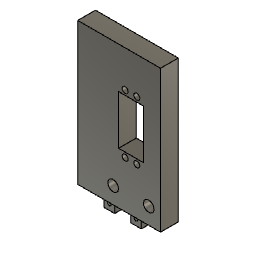
servo_side_stand_2 v20 (Autodesk Fusion 360 design; units mm, degrees)
Autodesk Fusion 360 part; units mm, degrees
note: some values were not read from the file. Set by a fixed rule: which sketch regions a step uses.
sketch "Sketch1" plane through (0, 0, 0) normal (0, 0, 1) x (1, 0, 0)
  line L0 (45, -7.5) -> (-45, -7.5) construction
  line L1 (-45, -7.5) -> (-45, 7.5) construction
  line L2 (-45, 7.5) -> (45, 7.5) construction
  line L3 (45, 7.5) -> (45, -7.5) construction
  line L4 (45, -7.5) -> (-45, 7.5) construction
  line L5 (-45, -7.5) -> (45, 7.5) construction
  line L6 (0, -7.5) -> (45, 7.5) construction
  line L7 (-45, 7.5) -> (0, -7.5) construction
  line L8 (4.5, -3.25) -> (-4.5, -3.25)
  line L9 (-4.5, -3.25) -> (-4.5, 3.25)
  line L10 (-4.5, 3.25) -> (4.5, 3.25)
  line L11 (4.5, 3.25) -> (4.5, -3.25)
  line L12 (4.5, -3.25) -> (-4.5, 3.25) construction
  line L13 (-4.5, -3.25) -> (4.5, 3.25) construction
  line L14 (-27, -3.25) -> (-18, -3.25)
  line L15 (-18, -3.25) -> (-18, 3.25)
  line L16 (-18, 3.25) -> (-27, 3.25)
  line L17 (-27, 3.25) -> (-27, -3.25)
  line L18 (-27, -3.25) -> (-18, 3.25) construction
  line L19 (-18, -3.25) -> (-27, 3.25) construction
  point P0 (22.5, 0)
  point P1 (-22.5, 0)
  dimension "d1" = 90
  dimension "d2" = 15
  dimension "d3" = 9
  dimension "d4" = 9
  dimension "d7" = 6.5
  dimension "d8" = 6.5
  constraint horizontal L0
  constraint perpendicular L0 L1
  constraint parallel L0 L2
  constraint parallel L1 L3
  constraint coincident L4 origin
  constraint coincident L5 origin
  constraint midpoint L0 L6.start
  constraint horizontal L8
  constraint perpendicular L8 L9
  constraint parallel L8 L10
  constraint parallel L9 L11
  constraint coincident L12 origin
  constraint coincident L13 origin
  constraint midpoint L6 P0
  constraint horizontal L14
  constraint perpendicular L14 L15
  constraint parallel L14 L16
  constraint parallel L15 L17
  constraint coincident L18 P1
  constraint coincident L19 P1
  constraint midpoint L7 P1
  measures "d1" distance of L0.start L0.end
  measures "d2" distance of L0.end L1.end
  measures "d3" distance of L14.start L14.end
  measures "d4" distance of L8.start L8.end
  measures "d7" distance of L8.start L10.end
  measures "d8" distance of L14.end L15.end
extrude "Extrude1" add sketch "Sketch1" along normal blind 10 makes body 1 at (-21, 3.25, 3.3333) makes body 2 at (-1.5, 3.25, 3.3333)
sketch "Sketch2" plane through (0, 0, 10) normal (0, 0, 1) x (-1, 0, 0)
  line L0 (45, 7.5) -> (-45, 7.5)
  line L1 (-45, 7.5) -> (-45, -7.5)
  line L2 (-45, -7.5) -> (45, -7.5)
  line L3 (45, -7.5) -> (45, 7.5)
  line L4 (45, 7.5) -> (-45, -7.5) construction
  line L5 (-45, 7.5) -> (45, -7.5) construction
  line L6 (27, -3.25) -> (27, 3.25)
  line L7 (27, 3.25) -> (18, 3.25)
  line L8 (18, 3.25) -> (18, -3.25)
  line L9 (18, -3.25) -> (27, -3.25)
  line L10 (-4.5, -3.25) -> (4.5, -3.25)
  line L11 (4.5, -3.25) -> (4.5, 3.25)
  line L12 (4.5, 3.25) -> (-4.5, 3.25)
  line L13 (-4.5, 3.25) -> (-4.5, -3.25)
  dimension "d11" = 90
  dimension "d12" = 15
  constraint horizontal L0
  constraint perpendicular L0 L1
  constraint parallel L0 L2
  constraint parallel L1 L3
  constraint coincident L4 origin
  constraint coincident L5 origin
  measures "d11" distance of L0.start L0.end
  measures "d12" distance of L0.start L2.end
extrude "Extrude2" add sketch "Sketch2" along normal blind 120 contours L0 L1 L2 L3 | L6 L7 L8 L9 | L10 L11 L12 L13 bodies 1 2
sketch "Sketch3" plane through (0, -7.5, 0) normal (0, -1, 0) x (1, 0, 0)
  line L0 (-45, 10) -> (45, 10)
  line L1 (45, 10) -> (45, 130)
  line L2 (45, 130) -> (-45, 130)
  line L3 (-45, 130) -> (-45, 10)
  line L4 (0, 10) -> (0, 74.4) construction
  line L5 (10.5, 53.65) -> (-10.5, 53.65)
  line L6 (-10.5, 53.65) -> (-10.5, 95.15)
  line L7 (-10.5, 95.15) -> (10.5, 95.15)
  line L8 (10.5, 95.15) -> (10.5, 53.65)
  line L9 (10.5, 53.65) -> (-10.5, 95.15) construction
  line L10 (-10.5, 53.65) -> (10.5, 95.15) construction
  line L11 (10, 49.65) -> (-10, 49.65) construction
  line L12 (-10, 49.65) -> (-10, 99.15) construction
  line L13 (-10, 99.15) -> (10, 99.15) construction
  line L14 (10, 99.15) -> (10, 49.65) construction
  line L15 (10, 49.65) -> (-10, 99.15) construction
  line L16 (-10, 49.65) -> (10, 99.15) construction
  circle A0 centre (4.925, 99.15) radius 2.5
  line L17 (0, 99.15) -> (0, 74.4) construction
  circle A1 centre (-4.925, 99.15) radius 2.5
  line L18 (0, 74.4) -> (10, 74.4) construction
  circle A2 centre (-4.925, 49.65) radius 2.5
  circle A3 centre (4.925, 49.65) radius 2.5
  point P0 (0, 74.4)
  point P1 (0, 74.4)
  point P2 (4.925, 99.15)
  dimension "d15" = 64.4
  dimension "d16" = 41.5
  dimension "d17" = 21
  dimension "d18" = 20
  dimension "d19" = 49.5
  dimension "d20" = 4.925
  dimension "d21" = 5
  constraint midpoint L0 L4.start
  constraint perpendicular L0 L4
  constraint horizontal L5
  constraint perpendicular L5 L6
  constraint parallel L5 L7
  constraint parallel L6 L8
  constraint coincident L9 P1
  constraint coincident L10 P1
  constraint coincident P1 P0
  constraint horizontal L11
  constraint perpendicular L11 L12
  constraint parallel L11 L13
  constraint parallel L12 L14
  constraint coincident L15 P1
  constraint coincident L16 P1
  constraint coincident L13 P2
  constraint coincident P2 A0.centre
  constraint symmetric A0 L17 A1
  constraint midpoint L14 L18.end
  constraint symmetric A0 L18 A3
  constraint symmetric A1 L18 A2
  measures "d15" distance of L4.start P1
  measures "d16" distance of L5.end L6.end
  measures "d17" distance of L6.end L7.end
  measures "d18" distance of L12.end L13.end
  measures "d19" distance of L11.start L13.end
  measures "d20" distance of P2 L17.start
  measures "d21" diameter of A0
extrude "Extrude3" cut sketch "Sketch3" against normal blind 15 contours L5 L6 L7 L8 | A0 | A1 | A2 | A3 bodies 1
sketch "Sketch4" plane through (0, -3.25, 0) normal (0, -1, 0) x (1, 0, 0)
  line L0 (-27, 0) -> (-18, 0)
  line L1 (-18, 0) -> (-18, 10)
  line L2 (-18, 10) -> (-27, 10)
  line L3 (-27, 10) -> (-27, 0)
  line L4 (-27, 10) -> (-18, 0) construction
  circle A0 centre (-22.5, 5) radius 1.5
  line L5 (-5, 10) -> (5, 0) construction
  line L6 (17.5, 10) -> (27.5, 0) construction
  circle A1 centre (0, 5) radius 1.5
  circle A2 centre (22.5, 5) radius 1.5
  dimension "d24" = 3
  dimension "d25" = 3
  dimension "d26" = 3
  constraint coincident L2.end L3.start
  constraint coincident L0.end L1.start
  constraint midpoint L4 A0.centre
  constraint midpoint L5 A1.centre
  constraint midpoint L6 A2.centre
  measures "d24" diameter of A0
  measures "d25" diameter of A1
  measures "d26" diameter of A2
extrude "Extrude4" cut sketch "Sketch4" against normal blind 10 contours A0 | A1 | A2 bodies 1
extrude "Extrude5" cut 1 faces at (45, -2.5, 50) along direction (-1, 0, 0) blind 20 on bodies 1 bodies 1
sketch "Sketch5" plane through (0, -7.5, 0) normal (0, -1, 0) x (1, 0, 0)
  line L0 (25, 10) -> (25, 130)
  line L1 (25, 130) -> (-45, 130)
  line L2 (-45, 130) -> (-45, 10)
  line L3 (-45, 10) -> (25, 10)
  circle A0 centre (4.925, 99.15) radius 2.5
  circle A1 centre (-4.925, 99.15) radius 2.5
  circle A2 centre (-4.925, 49.65) radius 2.5
  line L4 (-10.5, 53.65) -> (-10.5, 95.15)
  line L5 (-10.5, 95.15) -> (10.5, 95.15)
  line L6 (10.5, 95.15) -> (10.5, 53.65)
  line L7 (10.5, 53.65) -> (-10.5, 53.65)
  circle A3 centre (4.925, 49.65) radius 2.5
  line L8 (0, 10) -> (15, 10) construction
  line L9 (0, 10) -> (-15, 10) construction
  line L10 (-15, 10) -> (-15, 24) construction
  line L11 (15, 10) -> (15, 24) construction
  circle A4 centre (15, 24) radius 4.5
  circle A5 centre (-15, 24) radius 4.5
  dimension "d31" = 14
  dimension "d32" = 14
  dimension "d33" = 15
  dimension "d34" = 15
  dimension "d35" = 9
  dimension "d36" = 9
  constraint coincident L3 L8.start
  constraint coincident L3 L8.end
  constraint perpendicular L0 L8
  constraint coincident L3 L9.end
  constraint perpendicular L0 L9
  constraint perpendicular L3 L10
  constraint perpendicular L8 L11
  constraint coincident L11.end A4.centre
  constraint coincident L10.end A5.centre
  measures "d31" distance of L8.end L11.end
  measures "d32" distance of L9.end L10.end
  measures "d33" distance of L8.start L9.end
  measures "d34" distance of L8.start L8.end
  measures "d35" diameter of A4
  measures "d36" diameter of A5
extrude "Extrude6" cut sketch "Sketch5" against normal up to surface (15 mm away) contours A4 | A5 bodies 1
